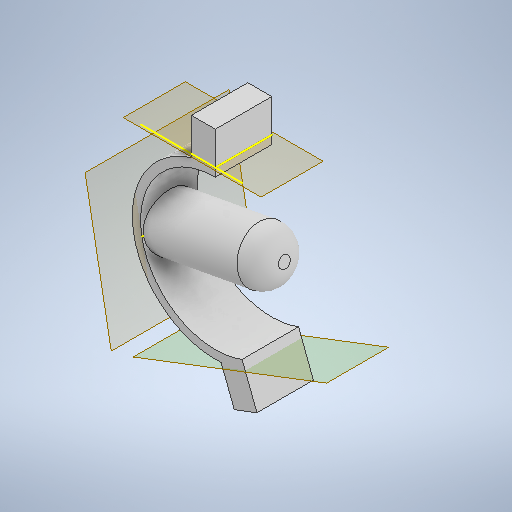
# Autodesk Inventor part: Clip1
Saved by Autodesk Inventor 2025 (Build 290162010, 162A)
## iProperties
Created: 2026-02-12
Part Number: Clip1
Material: Generic
Document SubType Name: Modeling
Designer: 925699
Density: 1 g/cm^3
Appearance: Default
Author: 925699
Autodesk Inventor part; units mm, degrees
ref_plane "YZ Plane" through (0, 0, 0) normal (1, 0, 0) x (0, 1, 0)
ref_plane "XZ Plane" through (0, 0, 0) normal (0, 1, 0) x (-1, 0, 0)
sketch "Sketch1" plane through (0, 0, 0) normal (0, 0, 1) x (1, 0, 0)
  arc A0 (0, 12.7) -> (4.541, -11.8604) centre (0, 0) ccw
  arc A1 (0, 11.43) -> (4.0869, -10.6744) centre (0, 0) ccw
  line L0 (0, 11.43) -> (0, 12.7)
  line L1 (4.541, -11.8604) -> (4.0869, -10.6744)
  dimension "d0" = 25.4
  dimension "d1" = 22.86
  constraints: 4 end point, 4 point on circle, 2 centre point, 2 coincident, 1 vertical
  measures "d0" diameter of A0
  measures "d1" diameter of A1
extrude "Extrusion1" add sketch "Sketch1" along normal blind 8.636
ref_plane "Work Plane1" through (0, 0, 0) normal (0.1818, -0.9833, 0) x (0, 0, -1)
sketch "Sketch2" plane through (0, 0, 0) normal (0.1818, -0.9833, 0) x (0, 0, -1)
  line L0 (-8.636, -11.43) -> (0, -11.43) projected
  point P0 (0, 0)
  point P1 (-4.318, -11.43)
  constraints: 1 midpoint
ref_plane "Work Plane2" through (-11.2395, -2.0781, 4.318) normal (0.9833, 0.1818, 0) x (-0.1818, 0.9833, 0)
sketch "Sketch3" plane through (-11.2395, -2.0781, 4.318) normal (0.9833, 0.1818, 0) x (-0.1818, 0.9833, 0)
  circle A0 centre (0, 0) radius 4.064
  point P0 (0, -4.318)
  dimension "d4" = 8.128
  constraints: 1 centre point
  measures "d4" diameter of A0
extrude "Extrusion2" add sketch "Sketch3" along normal blind 17.78
fillet "Fillet1" radius 3.175 1 edges at (6.983, -2.8418, 4.318)
ref_plane "Work Plane3" through (0, 12.7, 0) normal (0, 1, 0) x (-1, 0, 0)
sketch "Sketch4" plane through (0, 12.7, 0) normal (0, 1, 0) x (-1, 0, 0)
  line L0 (0, 0) -> (0, 8.636) projected
  line L1 (-4.0869, 8.636) -> (11.43, 8.636) projected
  line L2 (0, 0) -> (3.6716, 0)
  line L3 (3.6716, 0) -> (3.6716, 8.636)
  line L4 (3.6716, 8.636) -> (0, 8.636)
  line L5 (0, 8.636) -> (0, 0)
  constraints: 8 end point, 2 parallel, 1 horizontal, 1 midpoint, 1 perpendicular
extrude "Extrusion3" add sketch "Sketch4" along normal blind 5.08 and the other way blind 0.9525
ref_plane "Work Plane4" through (4.541, -11.8604, 0) normal (0.3576, -0.9339, 0) x (0.9339, 0.3576, 0)
sketch "Sketch5" plane through (4.541, -11.8604, 0) normal (0.3576, -0.9339, 0) x (0.9339, 0.3576, 0)
  line L0 (-3.7062, 0) -> (-3.7062, 8.66)
  line L1 (-3.7062, 0) -> (0, 0)
  line L2 (0, 0) -> (0, 8.636)
  line L3 (0, 8.636) -> (-3.7062, 8.636)
  line L4 (-3.7062, 8.636) -> (-3.7062, 0)
  line L5 (0.9182, 8.636) -> (-12.7, 8.636) projected
  line L6 (0, 0) -> (0, 8.636) projected
  line L7 (0.9182, 0) -> (-12.7, 0) projected
  point P0 (-3.7062, 8.636)
  dimension "d12" = 0
  dimension "d13" = 0
  dimension "d14" = 0
  constraints: 10 end point, 2 parallel, 1 horizontal, 1 perpendicular
  measures "d12" distance between parallel lines of L3 L5
  measures "d13" distance between parallel lines of L6 L2
  measures "d14" distance between parallel lines of L7 L1
extrude "Extrusion4" add sketch "Sketch5" along normal blind 5.08 and the other way blind 1.016
body "Solid1"
